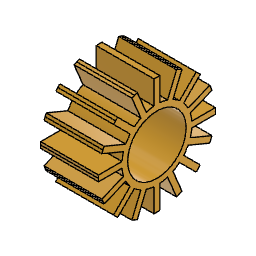
WaterMillWheelf3 (Autodesk Fusion 360 design; units mm, degrees)
Autodesk Fusion 360 part; units mm, degrees
sketch "Sketch2" plane through (0, 0, 0) normal (1, 0, 0) x (0, 1, 0)
  circle A0 centre (0, 0) radius 30
  circle A1 centre (0, 0) radius 25
  line L0 (-30, 0) -> (30, 0) construction
  line L1 (0, 45) -> (0, -45) construction
  line L2 (-2.5, 29.8957) -> (-2.5, 50)
  line L3 (-2.5, 50) -> (0, 50)
  line L4 (2.5, 29.8957) -> (2.5, 50)
  line L5 (2.5, 50) -> (0, 50)
  line L6 (-13.7503, 26.6633) -> (-21.4439, 45.2373)
  line L7 (-16.8245, 47.1507) -> (-19.1342, 46.194)
  line L8 (-9.1309, 28.5767) -> (-16.8245, 47.1507)
  line L9 (-21.4439, 45.2373) -> (-19.1342, 46.194)
  line L10 (-22.9072, 19.3717) -> (-37.1231, 33.5876)
  line L11 (-33.5876, 37.1231) -> (-35.3553, 35.3553)
  line L12 (-19.3717, 22.9072) -> (-33.5876, 37.1231)
  line L13 (-37.1231, 33.5876) -> (-35.3553, 35.3553)
  line L14 (-28.5767, 9.1309) -> (-47.1507, 16.8245)
  line L15 (-45.2373, 21.4439) -> (-46.194, 19.1342)
  line L16 (-26.6633, 13.7503) -> (-45.2373, 21.4439)
  line L17 (-47.1507, 16.8245) -> (-46.194, 19.1342)
  line L18 (-29.8957, -2.5) -> (-50, -2.5)
  line L19 (-50, 2.5) -> (-50, 0)
  line L20 (-29.8957, 2.5) -> (-50, 2.5)
  line L21 (-50, -2.5) -> (-50, 0)
  line L22 (-26.6633, -13.7503) -> (-45.2373, -21.4439)
  line L23 (-47.1507, -16.8245) -> (-46.194, -19.1342)
  line L24 (-28.5767, -9.1309) -> (-47.1507, -16.8245)
  line L25 (-45.2373, -21.4439) -> (-46.194, -19.1342)
  line L26 (-19.3717, -22.9072) -> (-33.5876, -37.1231)
  line L27 (-37.1231, -33.5876) -> (-35.3553, -35.3553)
  line L28 (-22.9072, -19.3717) -> (-37.1231, -33.5876)
  line L29 (-33.5876, -37.1231) -> (-35.3553, -35.3553)
  line L30 (-9.1309, -28.5767) -> (-16.8245, -47.1507)
  line L31 (-21.4439, -45.2373) -> (-19.1342, -46.194)
  line L32 (-13.7503, -26.6633) -> (-21.4439, -45.2373)
  line L33 (-16.8245, -47.1507) -> (-19.1342, -46.194)
  line L34 (2.5, -29.8957) -> (2.5, -50)
  line L35 (-2.5, -50) -> (0, -50)
  line L36 (-2.5, -29.8957) -> (-2.5, -50)
  line L37 (2.5, -50) -> (0, -50)
  line L38 (13.7503, -26.6633) -> (21.4439, -45.2373)
  line L39 (16.8245, -47.1507) -> (19.1342, -46.194)
  line L40 (9.1309, -28.5767) -> (16.8245, -47.1507)
  line L41 (21.4439, -45.2373) -> (19.1342, -46.194)
  line L42 (22.9072, -19.3717) -> (37.1231, -33.5876)
  line L43 (33.5876, -37.1231) -> (35.3553, -35.3553)
  line L44 (19.3717, -22.9072) -> (33.5876, -37.1231)
  line L45 (37.1231, -33.5876) -> (35.3553, -35.3553)
  line L46 (28.5767, -9.1309) -> (47.1507, -16.8245)
  line L47 (45.2373, -21.4439) -> (46.194, -19.1342)
  line L48 (26.6633, -13.7503) -> (45.2373, -21.4439)
  line L49 (47.1507, -16.8245) -> (46.194, -19.1342)
  line L50 (29.8957, 2.5) -> (50, 2.5)
  line L51 (50, -2.5) -> (50, 0)
  line L52 (29.8957, -2.5) -> (50, -2.5)
  line L53 (50, 2.5) -> (50, 0)
  line L54 (26.6633, 13.7503) -> (45.2373, 21.4439)
  line L55 (47.1507, 16.8245) -> (46.194, 19.1342)
  line L56 (28.5767, 9.1309) -> (47.1507, 16.8245)
  line L57 (45.2373, 21.4439) -> (46.194, 19.1342)
  line L58 (19.3717, 22.9072) -> (33.5876, 37.1231)
  line L59 (37.1231, 33.5876) -> (35.3553, 35.3553)
  line L60 (22.9072, 19.3717) -> (37.1231, 33.5876)
  line L61 (33.5876, 37.1231) -> (35.3553, 35.3553)
  line L62 (9.1309, 28.5767) -> (16.8245, 47.1507)
  line L63 (21.4439, 45.2373) -> (19.1342, 46.194)
  line L64 (13.7503, 26.6633) -> (21.4439, 45.2373)
  line L65 (16.8245, 47.1507) -> (19.1342, 46.194)
  dimension "d1" = 60
  dimension "d2" = 50
  dimension "d4" = 2.5
  dimension "d5" = 50
  dimension "d7" = 360
  constraint coincident A0.centre A1.centre
  constraint coincident A0 L0.start
  constraint coincident A0 L0.end
  constraint perpendicular L0 L1
  constraint coincident A0 L2.start
  constraint vertical L2
  constraint perpendicular L2 L3
  constraint symmetric L1 L2.start L4.start
  constraint symmetric L1 L2.end L4.end
  constraint symmetric L1 L3.end L5.end
  measures "d1" diameter of A0
  measures "d2" diameter of A1
  measures "d4" distance of L1 L2
  measures "d5" distance of A0.centre L3
extrude "Extrude1" add sketch "Sketch2" along normal blind 49.5
